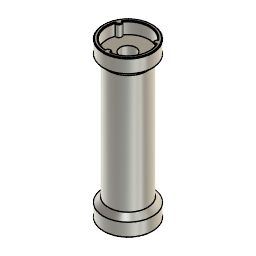
spool roller (Autodesk Fusion 360 design; units mm, degrees)
Autodesk Fusion 360 part; units mm, degrees
sketch "Sketch1" plane through (0, 0, 0) normal (0, 0, 1) x (1, 0, 0)
  circle A0 centre (0, 0) radius 12.5
  circle A1 centre (0, 0) radius 14.5
  dimension "d1" = 25
  dimension "d2" = 2
  constraint coincident A0.centre A1.centre
  measures "d1" diameter of A0
extrude "Extrude1" add sketch "Sketch1" along normal blind 7
sketch "Sketch2" plane through (0, 0, 0) normal (0, 0, -1) x (1, 0, 0)
  circle A0 centre (0, 0) radius 12.5
  circle A1 centre (0, 0) radius 14.5
extrude "Extrude2" add sketch "Sketch2" along normal blind 1 contours A0 | A1
sketch "Sketch3" plane through (0, 0, -1) normal (0, 0, -1) x (1, 0, 0)
  circle A0 centre (0, 0) radius 14.5
  circle A1 centre (0, 0) radius 4.6
  dimension "d7" = 9.2
  constraint coincident A0.centre A1.centre
  measures "d7" diameter of A1
extrude "Extrude3" cut sketch "Sketch3" against normal blind 1 contours A1
sketch "Sketch4" plane through (0, 0, -1) normal (0, 0, -1) x (1, 0, 0)
  circle A0 centre (0, 0) radius 4.6
  circle A1 centre (0, 0) radius 14.5
  circle A2 centre (0, 0) radius 11.5
  dimension "d10" = 23
  constraint coincident A0.centre A1.centre
  measures "d10" diameter of A2
extrude "Extrude4" add sketch "Sketch4" along normal blind 38 contours A2
chamfer "Chamfer1" distance 3 angle 45 1 edges at (-10.7218, -4.1586, -1)
sketch "Sketch5" plane through (0, 0, 7) normal (0, 0, 1) x (-1, 0, 0)
  circle A0 centre (0, 0) radius 12.5
  circle A1 centre (0, 0) radius 14.5
  circle A2 centre (0, 0) radius 10.85
  circle A3 centre (-0.6001, 12.4856) radius 1.65
  dimension "d16" = 21.7
  constraint coincident A0.centre A1.centre
  constraint coincident A0 A3.centre
  constraint tangent A2 A3
  measures "d16" diameter of A2
extrude "Extrude5" add sketch "Sketch5" against normal blind 7 contours A0 A3 picked at (-0.5733, 11.9282)
pattern_circular "C-Pattern1" count 3 over 360 about axis through (0, 0, -39) along (0, 0, 1) of "Extrude5"
mirror "Mirror2" about plane through (0, 0, -39) normal (0, 0, -1) of bodies 1 merged
chamfer "Chamfer2" distance 0.4 angle 45 1 faces at (10.941, 7.1918, 7)
chamfer "Chamfer3" distance 0.4 angle 45 1 faces at (10.941, 7.1918, -85)
